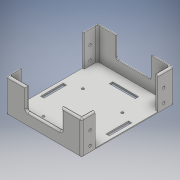
# Autodesk Inventor part: my_body
Saved by Autodesk Inventor 2017.2 (Build 212231000, 231)
## iProperties
Part Number: my_body
Material: Типовые
Document SubType Name: Modeling
Designer: creat
Density: 1 g/cm^3
Appearance: По умолчанию
Author: creat
Autodesk Inventor part; units mm, degrees
ref_plane "YZ Plane" through (0, 0, 0) normal (1, 0, 0) x (0, 1, 0)
ref_plane "XZ Plane" through (0, 0, 0) normal (0, 1, 0) x (-1, 0, 0)
ref_plane "XY Plane" through (0, 0, 0) normal (0, 0, 1) x (1, 0, 0)
sketch "Эскиз1" plane through (0, 0, 0) normal (0, 0, 1) x (1, 0, 0)
  line L0 (0, 12) -> (86, 12)
  line L1 (88, 10) -> (88, -96)
  line L2 (86, -98) -> (0, -98)
  line L3 (-2, -96) -> (-2, 10)
  line L4 (86, -98) -> (86, -96)
  line L5 (86, -96) -> (88, -96)
  arc A0 (-2, -96) -> (0, -98) centre (0, -96) ccw
  arc A1 (0, 12) -> (-2, 10) centre (0, 10) ccw
  arc A2 (88, 10) -> (86, 12) centre (86, 10) ccw
  arc A3 (86, -98) -> (88, -96) centre (86, -96) ccw
  point P0 (0, 0)
  point P1 (88, -98)
  point P2 (88, 12)
  point P3 (-2, -98)
  dimension "d0" = 90
  dimension "d1" = 110
  dimension "d4" = 2
  dimension "d5" = 2
  dimension "d10" = 2
  constraints: 12 end point, 8 point on circle, 8 tangent, 6 point on line, 4 centre point, 3 equal radius, 2 parallel, 1 horizontal, 1 perpendicular
  measures "d0" distance of point (88, -98) point (-2, -98)
  measures "d1" distance of point (88, 12) point (88, -98)
  measures "d4" distance of L4.end L5.end
  measures "d5" distance of L4.start L4.end
  measures "d10" radius of A0
extrude "Выдавливание1" add sketch "Эскиз1" along normal blind 40
sketch "Эскиз2" plane through (0, 0, 40) normal (0, 0, 1) x (1, 0, 0)
  line L0 (2, 9) -> (83.6156, 9)
  line L1 (85.6156, 7) -> (85.6156, -93.4907)
  line L2 (83.6156, -95.4907) -> (2, -95.4907)
  line L3 (0, -93.4907) -> (0, 7)
  arc A0 (83.6156, -95.4907) -> (85.6156, -93.4907) centre (83.6156, -93.4907) ccw
  arc A1 (0, -93.4907) -> (2, -95.4907) centre (2, -93.4907) ccw
  circle A2 centre (23.0817, -76.0567) radius 1.3003
  circle A3 centre (18, -24) radius 1.4794
  circle A4 centre (66.2724, -25.2355) radius 1.3051
  circle A5 centre (50.9777, -76.0071) radius 1.4879
  arc A6 (85.6156, 7) -> (83.6156, 9) centre (83.6156, 7) ccw
  arc A7 (2, 9) -> (0, 7) centre (2, 7) ccw
  point P0 (0, 0)
  point P1 (85.6156, -95.4907)
  point P2 (85.6156, 7.0453)
  point P3 (0, -95.4907)
  point P4 (85.6156, 9)
  point P5 (85.6156, -1.9999)
  dimension "d37" = 2
  constraints: 8 centre point, 8 end point, 8 point on circle, 8 point on line, 7 tangent, 1 equal radius, 1 horizontal, 1 parallel, 1 perpendicular
  measures "d37" radius of A6
extrude "Выдавливание2" cut sketch "Эскиз2" against normal blind 38 contours L0 A6 L1 A0 L2 A1 L3 A7 | A2 | A3 | A4 | A5
sketch "Эскиз3" plane through (88, -96, 0) normal (1, 0, 0) x (0, 0, -1)
  circle A0 centre (-23.5, 8) radius 1.5
  circle A1 centre (-7.5, 8) radius 1.5
  circle A2 centre (-23.5, 96) radius 1.5
  circle A3 centre (-7.5, 96) radius 1.5
  point P0 (0, 96)
  dimension "d15" = 3
  dimension "d16" = 3
  dimension "d17" = 3
  dimension "d18" = 3
  constraints: 4 centre point
  measures "d15" diameter of A0
  measures "d16" diameter of A1
  measures "d17" diameter of A2
  measures "d18" diameter of A3
extrude "Выдавливание3" cut sketch "Эскиз3" against normal blind 98.25
sketch "Эскиз4" plane through (0, -98, 0) normal (0, -1, 0) x (1, 0, 0)
  line L0 (22, 40) -> (64, 40)
  line L1 (64, 40) -> (64, 17)
  line L2 (62, 15) -> (24, 15)
  line L3 (22, 17) -> (22, 40)
  arc A0 (22, 17) -> (24, 15) centre (24, 17) ccw
  arc A1 (62, 15) -> (64, 17) centre (62, 17) ccw
  point P0 (0, 0)
  point P1 (64, 15)
  point P2 (22, 15)
  dimension "d21" = 42
  dimension "d22" = 25
  dimension "d25" = 2
  constraints: 8 end point, 4 point on circle, 4 point on line, 4 tangent, 2 centre point, 2 parallel, 1 equal radius, 1 horizontal, 1 perpendicular
  measures "d21" distance of point (64, 15) point (22, 15)
  measures "d22" distance of L0.end point (64, 15)
  measures "d25" radius of A0
extrude "Выдавливание4" cut sketch "Эскиз4" against normal blind 116.5
fillet "Сопряжение1" radius 2 20 edges at (-1.4142, -97.4142, 40) (-2, -43, 40) (-1.4142, 11.4142, 40) (11, 12, 40) (11, -98, 40) (22.5858, -98, 15.5858) (43, -98, 15) (63.4142, -98, 15.5858) (64, -98, 28.5) (22, -98, 28.5) (87.4142, -97.4142, 40) (88, -43, 40) (87.4142, 11.4142, 40) (75, 12, 40) (75, -98, 40) (63.4142, 12, 15.5858) (64, 12, 28.5) (22.5858, 12, 15.5858) (22, 12, 28.5) (43, 12, 15)
sketch "Эскиз5" plane through (-2, -96, 0) normal (-1, 0, 0) x (0, 0, 1)
  line L0 (9, 91) -> (40, 91)
  line L1 (40, 91) -> (40, 13)
  line L2 (40, 13) -> (9, 13)
  line L3 (7, 15) -> (7, 89)
  arc A0 (9, 91) -> (7, 89) centre (9, 89) ccw
  arc A1 (7, 15) -> (9, 13) centre (9, 15) ccw
  point P0 (0, 96)
  dimension "d27" = 2
  constraints: 8 end point, 4 point on circle, 2 centre point, 2 parallel, 2 tangent, 1 equal radius, 1 horizontal, 1 perpendicular
  measures "d27" radius of A0
extrude "Выдавливание5" [suppressed]
fillet "Сопряжение2" radius 1 8 edges at (-1.4142, 11.4142, 0) (43, 12, 0) (87.4142, 11.4142, 0) (88, -43, 0) (87.4142, -97.4142, 0) (43, -98, 0) (-1.4142, -97.4142, 0) (-2, -43, 0)
fillet "Сопряжение3" [suppressed]
sketch "Эскиз6" plane through (0, 0, 0) normal (0, 0, -1) x (-1, 0, 0)
  line L0 (-2, -34) -> (-6, -34)
  line L1 (-6, -34) -> (-6, -61)
  line L2 (-6, -61) -> (-2, -61)
  line L3 (-2, -61) -> (-2, -34)
  line L4 (-80, -34) -> (-84, -34)
  line L5 (-84, -34) -> (-84, -61)
  line L6 (-84, -61) -> (-80, -61)
  line L7 (-80, -61) -> (-80, -34)
  line L8 (-27, -90) -> (-58, -90)
  line L9 (-58, -90) -> (-58, -94)
  line L10 (-58, -94) -> (-27, -94)
  line L11 (-27, -94) -> (-27, -90)
  line L12 (-30, -3) -> (-61, -3)
  line L13 (-61, -3) -> (-61, -7)
  line L14 (-61, -7) -> (-30, -7)
  line L15 (-30, -7) -> (-30, -3)
  point P0 (0, 0)
  constraints: 32 end point, 8 parallel, 4 horizontal, 4 perpendicular
extrude "Выдавливание6" cut sketch "Эскиз6" against normal blind 2.75
sketch "Эскиз7" plane through (0, 0, 2) normal (0, 0, 1) x (1, 0, 0)
  line L0 (69.5594, -14.0478) -> (69.7922, -14.1325)
  line L1 (70.1519, -14.5133) -> (70.2577, -14.7461)
  line L2 (70.0038, -14.3017) -> (70.1519, -14.5133)
  line L3 (69.7922, -14.1325) -> (70.0038, -14.3017)
  line L4 (70.3, -78.4776) -> (68.7765, -80.001)
  line L5 (69.2844, -14.0055) -> (69.5594, -14.0478)
  line L6 (17.9945, -14.0055) -> (69.2844, -14.0055)
  line L7 (17.7406, -14.0478) -> (17.9945, -14.0055)
  line L8 (17.5078, -14.1325) -> (17.7406, -14.0478)
  line L9 (17.2962, -14.3017) -> (17.5078, -14.1325)
  line L10 (17.127, -14.5133) -> (17.2962, -14.3017)
  line L11 (17.0423, -14.7461) -> (17.127, -14.5133)
  line L12 (17, -15) -> (17.0423, -14.7461)
  line L13 (17, -79.0066) -> (17, -15)
  line L14 (17.0423, -79.2605) -> (17, -79.0066)
  line L15 (17.127, -79.4932) -> (17.0423, -79.2605)
  line L16 (17.2962, -79.7048) -> (17.127, -79.4932)
  line L17 (17.5078, -79.8741) -> (17.2962, -79.7048)
  line L18 (17.7406, -79.9587) -> (17.5078, -79.8741)
  line L19 (17.9945, -80.001) -> (17.7406, -79.9587)
  line L20 (19.5391, -80.001) -> (17.9945, -80.001)
  line L21 (22.0782, -82.5401) -> (19.5391, -80.001)
  line L22 (54.8115, -82.5401) -> (22.0782, -82.5401)
  line L23 (57.3506, -80.001) -> (54.8115, -82.5401)
  line L24 (68.7765, -80.001) -> (57.3506, -80.001)
  line L25 (70.3, -15) -> (70.3, -78.4776)
  line L26 (70.2577, -14.7461) -> (70.3, -15)
  line L27 (66.1538, -29.2963) -> (66.1567, -29.3523)
  line L28 (66.1567, -29.3523) -> (66.1616, -29.4082)
  line L29 (66.1616, -29.4082) -> (66.1684, -29.4639)
  line L30 (66.1684, -29.4639) -> (66.1772, -29.5194)
  line L31 (66.1772, -29.5194) -> (66.1879, -29.5745)
  line L32 (66.1879, -29.5745) -> (66.2006, -29.6292)
  line L33 (66.2006, -29.6292) -> (66.2151, -29.6834)
  line L34 (66.2151, -29.6834) -> (66.2315, -29.7371)
  line L35 (66.2315, -29.7371) -> (66.2498, -29.7901)
  line L36 (66.2498, -29.7901) -> (66.2699, -29.8425)
  line L37 (66.2699, -29.8425) -> (66.2918, -29.8942)
  line L38 (66.2918, -29.8942) -> (66.3155, -29.9451)
  line L39 (66.3155, -29.9451) -> (66.341, -29.9951)
  line L40 (66.341, -29.9951) -> (66.3682, -30.0442)
  line L41 (66.3682, -30.0442) -> (66.3972, -30.0923)
  line L42 (66.3972, -30.0923) -> (66.4277, -30.1394)
  line L43 (66.4277, -30.1394) -> (66.4599, -30.1854)
  line L44 (66.4599, -30.1854) -> (66.4937, -30.2302)
  line L45 (66.4937, -30.2302) -> (66.529, -30.2738)
  line L46 (66.529, -30.2738) -> (66.5658, -30.3162)
  line L47 (66.5658, -30.3162) -> (66.6041, -30.3572)
  line L48 (66.6041, -30.3572) -> (66.6438, -30.3969)
  line L49 (66.6438, -30.3969) -> (66.6849, -30.4352)
  line L50 (66.6849, -30.4352) -> (66.7272, -30.472)
  line L51 (66.7272, -30.472) -> (66.7709, -30.5073)
  line L52 (66.7709, -30.5073) -> (66.8157, -30.5411)
  line L53 (66.8157, -30.5411) -> (66.8617, -30.5733)
  line L54 (66.8617, -30.5733) -> (66.9087, -30.6039)
  line L55 (66.9087, -30.6039) -> (66.9568, -30.6328)
  line L56 (66.9568, -30.6328) -> (67.0059, -30.66)
  line L57 (67.0059, -30.66) -> (67.056, -30.6855)
  line L58 (67.056, -30.6855) -> (67.1068, -30.7092)
  line L59 (67.1068, -30.7092) -> (67.1585, -30.7311)
  line L60 (67.1585, -30.7311) -> (67.2109, -30.7513)
  line L61 (67.2109, -30.7513) -> (67.264, -30.7695)
  line L62 (67.264, -30.7695) -> (67.3176, -30.7859)
  line L63 (67.3176, -30.7859) -> (67.3719, -30.8005)
  line L64 (67.3719, -30.8005) -> (67.4266, -30.8131)
  line L65 (67.4266, -30.8131) -> (67.4817, -30.8238)
  line L66 (67.4817, -30.8238) -> (67.5371, -30.8326)
  line L67 (67.5371, -30.8326) -> (67.5928, -30.8394)
  line L68 (67.5928, -30.8394) -> (67.6487, -30.8443)
  line L69 (67.6487, -30.8443) -> (67.7048, -30.8473)
  line L70 (67.7048, -30.8473) -> (67.7609, -30.8482)
  line L71 (67.7609, -30.8482) -> (67.8166, -30.8473)
  line L72 (67.8166, -30.8473) -> (67.8722, -30.8444)
  line L73 (67.8722, -30.8444) -> (67.9278, -30.8396)
  line L74 (67.9278, -30.8396) -> (67.9831, -30.8328)
  line L75 (67.9831, -30.8328) -> (68.0381, -30.8242)
  line L76 (68.0381, -30.8242) -> (68.0928, -30.8136)
  line L77 (68.0928, -30.8136) -> (68.1471, -30.8012)
  line L78 (68.1471, -30.8012) -> (68.201, -30.7868)
  line L79 (68.201, -30.7868) -> (68.2543, -30.7707)
  line L80 (68.2543, -30.7707) -> (68.307, -30.7527)
  line L81 (68.307, -30.7527) -> (68.3591, -30.7328)
  line L82 (68.3591, -30.7328) -> (68.4104, -30.7112)
  line L83 (68.4104, -30.7112) -> (68.461, -30.6878)
  line L84 (68.461, -30.6878) -> (68.5107, -30.6627)
  line L85 (68.5107, -30.6627) -> (68.5596, -30.6359)
  line L86 (68.5596, -30.6359) -> (68.6075, -30.6074)
  line L87 (68.6075, -30.6074) -> (68.6543, -30.5772)
  line L88 (68.6543, -30.5772) -> (68.7001, -30.5455)
  line L89 (68.7001, -30.5455) -> (68.7448, -30.5121)
  line L90 (68.7448, -30.5121) -> (68.7882, -30.4773)
  line L91 (68.7882, -30.4773) -> (68.8305, -30.441)
  line L92 (68.8305, -30.441) -> (68.8714, -30.4032)
  line L93 (68.8714, -30.4032) -> (68.9111, -30.364)
  line L94 (68.9111, -30.364) -> (68.9493, -30.3235)
  line L95 (68.9493, -30.3235) -> (68.9861, -30.2817)
  line L96 (68.9861, -30.2817) -> (69.0215, -30.2386)
  line L97 (69.0215, -30.2386) -> (69.0553, -30.1943)
  line L98 (69.0553, -30.1943) -> (69.0876, -30.1489)
  line L99 (69.0876, -30.1489) -> (69.1183, -30.1024)
  line L100 (69.1183, -30.1024) -> (69.1473, -30.0549)
  line L101 (69.1473, -30.0549) -> (69.1747, -30.0064)
  line L102 (69.1747, -30.0064) -> (69.2004, -29.9569)
  line L103 (69.2004, -29.9569) -> (69.2244, -29.9066)
  line L104 (69.2244, -29.9066) -> (69.2466, -29.8555)
  line L105 (69.2466, -29.8555) -> (69.267, -29.8037)
  line L106 (69.267, -29.8037) -> (69.2856, -29.7512)
  line L107 (69.2856, -29.7512) -> (69.3024, -29.698)
  line L108 (69.3024, -29.698) -> (69.3174, -29.6444)
  line L109 (69.3174, -29.6444) -> (69.3304, -29.5902)
  line L110 (69.3304, -29.5902) -> (69.3416, -29.5356)
  line L111 (69.3416, -29.5356) -> (69.3509, -29.4807)
  line L112 (69.3509, -29.4807) -> (69.3583, -29.4255)
  line L113 (69.3583, -29.4255) -> (69.3637, -29.37)
  line L114 (69.3637, -29.37) -> (69.3673, -29.3144)
  line L115 (69.3673, -29.3144) -> (69.3689, -29.2587)
  line L116 (69.3689, -29.2587) -> (69.3686, -29.203)
  line L117 (69.3686, -29.203) -> (69.3663, -29.1473)
  line L118 (69.3663, -29.1473) -> (69.3621, -29.0918)
  line L119 (66.1528, -29.2401) -> (66.1538, -29.2963)
  line L120 (69.356, -29.0364) -> (69.348, -28.9812)
  line L121 (69.348, -28.9812) -> (69.3381, -28.9264)
  line L122 (69.3381, -28.9264) -> (69.3263, -28.872)
  line L123 (69.3263, -28.872) -> (69.3126, -28.818)
  line L124 (69.3126, -28.818) -> (69.297, -28.7644)
  line L125 (69.297, -28.7644) -> (69.2796, -28.7115)
  line L126 (69.2796, -28.7115) -> (69.2604, -28.6592)
  line L127 (69.2604, -28.6592) -> (69.2394, -28.6076)
  line L128 (69.2394, -28.6076) -> (69.2166, -28.5568)
  line L129 (69.2166, -28.5568) -> (69.192, -28.5068)
  line L130 (69.192, -28.5068) -> (69.1658, -28.4576)
  line L131 (69.1658, -28.4576) -> (69.1378, -28.4094)
  line L132 (69.1378, -28.4094) -> (69.1082, -28.3622)
  line L133 (69.1082, -28.3622) -> (69.077, -28.3161)
  line L134 (69.077, -28.3161) -> (69.0442, -28.271)
  line L135 (69.0442, -28.271) -> (69.0098, -28.2272)
  line L136 (69.0098, -28.2272) -> (68.974, -28.1845)
  line L137 (68.974, -28.1845) -> (68.9367, -28.1431)
  line L138 (68.9367, -28.1431) -> (68.898, -28.103)
  line L139 (68.898, -28.103) -> (68.8579, -28.0643)
  line L140 (68.8579, -28.0643) -> (68.8165, -28.027)
  line L141 (68.8165, -28.027) -> (68.7739, -27.9912)
  line L142 (68.7739, -27.9912) -> (68.73, -27.9568)
  line L143 (68.73, -27.9568) -> (68.685, -27.924)
  line L144 (68.685, -27.924) -> (68.6388, -27.8928)
  line L145 (68.6388, -27.8928) -> (68.5916, -27.8632)
  line L146 (68.5916, -27.8632) -> (68.5434, -27.8353)
  line L147 (68.5434, -27.8353) -> (68.4943, -27.809)
  line L148 (68.4943, -27.809) -> (68.4442, -27.7845)
  line L149 (68.4442, -27.7845) -> (68.3934, -27.7617)
  line L150 (68.3934, -27.7617) -> (68.3418, -27.7406)
  line L151 (68.3418, -27.7406) -> (68.2895, -27.7214)
  line L152 (68.2895, -27.7214) -> (68.2366, -27.704)
  line L153 (68.2366, -27.704) -> (68.1831, -27.6884)
  line L154 (68.1831, -27.6884) -> (68.1291, -27.6748)
  line L155 (68.1291, -27.6748) -> (68.0746, -27.6629)
  line L156 (68.0746, -27.6629) -> (68.0198, -27.653)
  line L157 (68.0198, -27.653) -> (67.9647, -27.645)
  line L158 (67.9647, -27.645) -> (67.9093, -27.6389)
  line L159 (67.9093, -27.6389) -> (67.8537, -27.6347)
  line L160 (67.8537, -27.6347) -> (67.798, -27.6325)
  line L161 (67.798, -27.6325) -> (67.7423, -27.6321)
  line L162 (67.7423, -27.6321) -> (67.6866, -27.6338)
  line L163 (67.6866, -27.6338) -> (67.631, -27.6373)
  line L164 (67.631, -27.6373) -> (67.5756, -27.6428)
  line L165 (67.5756, -27.6428) -> (67.5203, -27.6501)
  line L166 (67.5203, -27.6501) -> (67.4654, -27.6594)
  line L167 (67.4654, -27.6594) -> (67.4108, -27.6706)
  line L168 (67.4108, -27.6706) -> (67.3567, -27.6837)
  line L169 (67.3567, -27.6837) -> (67.303, -27.6986)
  line L170 (67.303, -27.6986) -> (67.2499, -27.7154)
  line L171 (67.2499, -27.7154) -> (67.1973, -27.734)
  line L172 (67.1973, -27.734) -> (67.1455, -27.7544)
  line L173 (67.1455, -27.7544) -> (67.0944, -27.7767)
  line L174 (67.0944, -27.7767) -> (67.0441, -27.8006)
  line L175 (67.0441, -27.8006) -> (66.9947, -27.8263)
  line L176 (66.9947, -27.8263) -> (66.9461, -27.8537)
  line L177 (66.9461, -27.8537) -> (66.8986, -27.8828)
  line L178 (66.8986, -27.8828) -> (66.8521, -27.9135)
  line L179 (66.8521, -27.9135) -> (66.8067, -27.9457)
  line L180 (66.8067, -27.9457) -> (66.7624, -27.9796)
  line L181 (66.7624, -27.9796) -> (66.7193, -28.0149)
  line L182 (66.7193, -28.0149) -> (66.6775, -28.0517)
  line L183 (66.6775, -28.0517) -> (66.637, -28.09)
  line L184 (66.637, -28.09) -> (66.5978, -28.1296)
  line L185 (66.5978, -28.1296) -> (66.5601, -28.1706)
  line L186 (66.5601, -28.1706) -> (66.5237, -28.2128)
  line L187 (66.5237, -28.2128) -> (66.4889, -28.2563)
  line L188 (66.4889, -28.2563) -> (66.4556, -28.3009)
  line L189 (66.4556, -28.3009) -> (66.4238, -28.3467)
  line L190 (66.4238, -28.3467) -> (66.3937, -28.3936)
  line L191 (66.3937, -28.3936) -> (66.3652, -28.4415)
  line L192 (66.3652, -28.4415) -> (66.3383, -28.4903)
  line L193 (66.3383, -28.4903) -> (66.3132, -28.54)
  line L194 (66.3132, -28.54) -> (66.2898, -28.5906)
  line L195 (66.2898, -28.5906) -> (66.2682, -28.6419)
  line L196 (66.2682, -28.6419) -> (66.2484, -28.694)
  line L197 (66.2484, -28.694) -> (66.2304, -28.7467)
  line L198 (66.2304, -28.7467) -> (66.2142, -28.8001)
  line L199 (66.2142, -28.8001) -> (66.1999, -28.8539)
  line L200 (66.1999, -28.8539) -> (66.1874, -28.9082)
  line L201 (66.1874, -28.9082) -> (66.1769, -28.9629)
  line L202 (66.1769, -28.9629) -> (66.1682, -29.018)
  line L203 (66.1682, -29.018) -> (66.1615, -29.0733)
  line L204 (66.1615, -29.0733) -> (66.1567, -29.1288)
  line L205 (66.1567, -29.1288) -> (66.1538, -29.1844)
  line L206 (66.1538, -29.1844) -> (66.1528, -29.2401)
  line L207 (69.3621, -29.0918) -> (69.356, -29.0364)
  line L208 (50.9182, -80.001) -> (50.9192, -80.0572)
  line L209 (50.9192, -80.0572) -> (50.9221, -80.1132)
  line L210 (50.9221, -80.1132) -> (50.927, -80.1691)
  line L211 (50.927, -80.1691) -> (50.9338, -80.2248)
  line L212 (50.9338, -80.2248) -> (50.9426, -80.2803)
  line L213 (50.9426, -80.2803) -> (50.9533, -80.3354)
  line L214 (50.9533, -80.3354) -> (50.9659, -80.3901)
  line L215 (50.9659, -80.3901) -> (50.9805, -80.4443)
  line L216 (50.9805, -80.4443) -> (50.9969, -80.498)
  line L217 (50.9969, -80.498) -> (51.0152, -80.551)
  line L218 (51.0152, -80.551) -> (51.0353, -80.6034)
  line L219 (51.0353, -80.6034) -> (51.0572, -80.6551)
  line L220 (51.0572, -80.6551) -> (51.0809, -80.706)
  line L221 (51.0809, -80.706) -> (51.1064, -80.756)
  line L222 (51.1064, -80.756) -> (51.1336, -80.8051)
  line L223 (51.1336, -80.8051) -> (51.1625, -80.8532)
  line L224 (51.1625, -80.8532) -> (51.1931, -80.9003)
  line L225 (51.1931, -80.9003) -> (51.2253, -80.9462)
  line L226 (51.2253, -80.9462) -> (51.2591, -80.9911)
  line L227 (51.2591, -80.9911) -> (51.2944, -81.0347)
  line L228 (51.2944, -81.0347) -> (51.3312, -81.0771)
  line L229 (51.3312, -81.0771) -> (51.3695, -81.1181)
  line L230 (51.3695, -81.1181) -> (51.4092, -81.1578)
  line L231 (51.4092, -81.1578) -> (51.4503, -81.1961)
  line L232 (51.4503, -81.1961) -> (51.4926, -81.2329)
  line L233 (51.4926, -81.2329) -> (51.5362, -81.2682)
  line L234 (51.5362, -81.2682) -> (51.5811, -81.302)
  line L235 (51.5811, -81.302) -> (51.627, -81.3342)
  line L236 (51.627, -81.3342) -> (51.6741, -81.3648)
  line L237 (51.6741, -81.3648) -> (51.7222, -81.3937)
  line L238 (51.7222, -81.3937) -> (51.7713, -81.4209)
  line L239 (51.7713, -81.4209) -> (51.8213, -81.4464)
  line L240 (51.8213, -81.4464) -> (51.8722, -81.4701)
  line L241 (51.8722, -81.4701) -> (51.9239, -81.492)
  line L242 (51.9239, -81.492) -> (51.9763, -81.5122)
  line L243 (51.9763, -81.5122) -> (52.0294, -81.5304)
  line L244 (52.0294, -81.5304) -> (52.083, -81.5468)
  line L245 (52.083, -81.5468) -> (52.1372, -81.5614)
  line L246 (52.1372, -81.5614) -> (52.1919, -81.574)
  line L247 (52.1919, -81.574) -> (52.247, -81.5847)
  line L248 (52.247, -81.5847) -> (52.3025, -81.5935)
  line L249 (52.3025, -81.5935) -> (52.3582, -81.6003)
  line L250 (52.3582, -81.6003) -> (52.4141, -81.6052)
  line L251 (52.4141, -81.6052) -> (52.4702, -81.6082)
  line L252 (52.4702, -81.6082) -> (52.5263, -81.6091)
  line L253 (52.5263, -81.6091) -> (52.582, -81.6082)
  line L254 (52.582, -81.6082) -> (52.6376, -81.6053)
  line L255 (52.6376, -81.6053) -> (52.6931, -81.6005)
  line L256 (52.6931, -81.6005) -> (52.7484, -81.5937)
  line L257 (52.7484, -81.5937) -> (52.8035, -81.5851)
  line L258 (52.8035, -81.5851) -> (52.8582, -81.5745)
  line L259 (52.8582, -81.5745) -> (52.9125, -81.5621)
  line L260 (52.9125, -81.5621) -> (52.9664, -81.5477)
  line L261 (52.9664, -81.5477) -> (53.0197, -81.5316)
  line L262 (53.0197, -81.5316) -> (53.0724, -81.5136)
  line L263 (53.0724, -81.5136) -> (53.1245, -81.4937)
  line L264 (53.1245, -81.4937) -> (53.1758, -81.4721)
  line L265 (53.1758, -81.4721) -> (53.2264, -81.4487)
  line L266 (53.2264, -81.4487) -> (53.2761, -81.4236)
  line L267 (53.2761, -81.4236) -> (53.325, -81.3968)
  line L268 (53.325, -81.3968) -> (53.3728, -81.3683)
  line L269 (53.3728, -81.3683) -> (53.4197, -81.3381)
  line L270 (53.4197, -81.3381) -> (53.4655, -81.3064)
  line L271 (53.4655, -81.3064) -> (53.5101, -81.273)
  line L272 (53.5101, -81.273) -> (53.5536, -81.2382)
  line L273 (53.5536, -81.2382) -> (53.5959, -81.2019)
  line L274 (53.5959, -81.2019) -> (53.6368, -81.1641)
  line L275 (53.6368, -81.1641) -> (53.6764, -81.1249)
  line L276 (53.6764, -81.1249) -> (53.7147, -81.0844)
  line L277 (53.7147, -81.0844) -> (53.7515, -81.0426)
  line L278 (53.7515, -81.0426) -> (53.7868, -80.9995)
  line L279 (53.7868, -80.9995) -> (53.8207, -80.9552)
  line L280 (53.8207, -80.9552) -> (53.853, -80.9098)
  line L281 (53.853, -80.9098) -> (53.8836, -80.8633)
  line L282 (53.8836, -80.8633) -> (53.9127, -80.8158)
  line L283 (53.9127, -80.8158) -> (53.9401, -80.7673)
  line L284 (53.9401, -80.7673) -> (53.9658, -80.7178)
  line L285 (53.9658, -80.7178) -> (53.9898, -80.6675)
  line L286 (53.9898, -80.6675) -> (54.012, -80.6164)
  line L287 (54.012, -80.6164) -> (54.0324, -80.5646)
  line L288 (54.0324, -80.5646) -> (54.051, -80.5121)
  line L289 (54.051, -80.5121) -> (54.0678, -80.4589)
  line L290 (54.0678, -80.4589) -> (54.0827, -80.4053)
  line L291 (54.0827, -80.4053) -> (54.0958, -80.3511)
  line L292 (54.0958, -80.3511) -> (54.107, -80.2965)
  line L293 (54.107, -80.2965) -> (54.1163, -80.2416)
  line L294 (54.1163, -80.2416) -> (54.1237, -80.1864)
  line L295 (54.1237, -80.1864) -> (54.1291, -80.1309)
  line L296 (54.1291, -80.1309) -> (54.1327, -80.0753)
  line L297 (54.1327, -80.0753) -> (54.1343, -80.0196)
  line L298 (54.1343, -80.0196) -> (54.1339, -79.9639)
  line L299 (54.1339, -79.9639) -> (54.1317, -79.9082)
  line L300 (54.1317, -79.9082) -> (54.1275, -79.8527)
  line L301 (54.1275, -79.8527) -> (54.1214, -79.7973)
  line L302 (54.1214, -79.7973) -> (54.1134, -79.7421)
  line L303 (54.1134, -79.7421) -> (54.1035, -79.6873)
  line L304 (54.1035, -79.6873) -> (54.0917, -79.6329)
  line L305 (54.0917, -79.6329) -> (54.078, -79.5788)
  line L306 (54.078, -79.5788) -> (54.0624, -79.5253)
  line L307 (54.0624, -79.5253) -> (54.045, -79.4724)
  line L308 (54.045, -79.4724) -> (54.0258, -79.4201)
  line L309 (54.0258, -79.4201) -> (54.0048, -79.3685)
  line L310 (54.0048, -79.3685) -> (53.982, -79.3177)
  line L311 (53.982, -79.3177) -> (53.9574, -79.2677)
  line L312 (53.9574, -79.2677) -> (53.9312, -79.2185)
  line L313 (53.9312, -79.2185) -> (53.9032, -79.1703)
  line L314 (53.9032, -79.1703) -> (53.8736, -79.1231)
  line L315 (53.8736, -79.1231) -> (53.8424, -79.077)
  line L316 (53.8424, -79.077) -> (53.8096, -79.0319)
  line L317 (53.8096, -79.0319) -> (53.7752, -78.9881)
  line L318 (53.7752, -78.9881) -> (53.7394, -78.9454)
  line L319 (53.7394, -78.9454) -> (53.7021, -78.904)
  line L320 (53.7021, -78.904) -> (53.6634, -78.8639)
  line L321 (53.6634, -78.8639) -> (53.6233, -78.8252)
  line L322 (53.6233, -78.8252) -> (53.5819, -78.7879)
  line L323 (53.5819, -78.7879) -> (53.5393, -78.7521)
  line L324 (53.5393, -78.7521) -> (53.4954, -78.7177)
  line L325 (53.4954, -78.7177) -> (53.4503, -78.6849)
  line L326 (53.4503, -78.6849) -> (53.4042, -78.6537)
  line L327 (53.4042, -78.6537) -> (53.357, -78.6241)
  line L328 (53.357, -78.6241) -> (53.3088, -78.5962)
  line L329 (53.3088, -78.5962) -> (53.2596, -78.5699)
  line L330 (53.2596, -78.5699) -> (53.2096, -78.5453)
  line L331 (53.2096, -78.5453) -> (53.1588, -78.5225)
  line L332 (53.1588, -78.5225) -> (53.1072, -78.5015)
  line L333 (53.1072, -78.5015) -> (53.0549, -78.4823)
  line L334 (53.0549, -78.4823) -> (53.002, -78.4649)
  line L335 (53.002, -78.4649) -> (52.9485, -78.4493)
  line L336 (52.9485, -78.4493) -> (52.8945, -78.4356)
  line L337 (52.8945, -78.4356) -> (52.84, -78.4238)
  line L338 (52.84, -78.4238) -> (52.7852, -78.4139)
  line L339 (52.7852, -78.4139) -> (52.73, -78.4059)
  line L340 (52.73, -78.4059) -> (52.6747, -78.3998)
  line L341 (52.6747, -78.3998) -> (52.6191, -78.3956)
  line L342 (52.6191, -78.3956) -> (52.5634, -78.3934)
  line L343 (52.5634, -78.3934) -> (52.5077, -78.393)
  line L344 (52.5077, -78.393) -> (52.452, -78.3946)
  line L345 (52.452, -78.3946) -> (52.3964, -78.3982)
  line L346 (52.3964, -78.3982) -> (52.341, -78.4036)
  line L347 (52.341, -78.4036) -> (52.2857, -78.411)
  line L348 (52.2857, -78.411) -> (52.2308, -78.4203)
  line L349 (52.2308, -78.4203) -> (52.1762, -78.4315)
  line L350 (52.1762, -78.4315) -> (52.122, -78.4446)
  line L351 (52.122, -78.4446) -> (52.0684, -78.4595)
  line L352 (52.0684, -78.4595) -> (52.0152, -78.4763)
  line L353 (52.0152, -78.4763) -> (51.9627, -78.4949)
  line L354 (51.9627, -78.4949) -> (51.9109, -78.5153)
  line L355 (51.9109, -78.5153) -> (51.8598, -78.5376)
  line L356 (51.8598, -78.5376) -> (51.8095, -78.5615)
  line L357 (51.8095, -78.5615) -> (51.7601, -78.5872)
  line L358 (51.7601, -78.5872) -> (51.7115, -78.6146)
  line L359 (51.7115, -78.6146) -> (51.664, -78.6437)
  line L360 (51.664, -78.6437) -> (51.6175, -78.6744)
  line L361 (51.6175, -78.6744) -> (51.5721, -78.7066)
  line L362 (51.5721, -78.7066) -> (51.5278, -78.7405)
  line L363 (51.5278, -78.7405) -> (51.4847, -78.7758)
  line L364 (51.4847, -78.7758) -> (51.4429, -78.8126)
  line L365 (51.4429, -78.8126) -> (51.4024, -78.8509)
  line L366 (51.4024, -78.8509) -> (51.3632, -78.8905)
  line L367 (51.3632, -78.8905) -> (51.3254, -78.9315)
  line L368 (51.3254, -78.9315) -> (51.2891, -78.9737)
  line L369 (51.2891, -78.9737) -> (51.2543, -79.0172)
  line L370 (51.2543, -79.0172) -> (51.2209, -79.0618)
  line L371 (51.2209, -79.0618) -> (51.1892, -79.1076)
  line L372 (51.1892, -79.1076) -> (51.159, -79.1545)
  line L373 (51.159, -79.1545) -> (51.1305, -79.2024)
  line L374 (51.1305, -79.2024) -> (51.1037, -79.2512)
  line L375 (51.1037, -79.2512) -> (51.0786, -79.3009)
  line L376 (51.0786, -79.3009) -> (51.0552, -79.3515)
  line L377 (51.0552, -79.3515) -> (51.0336, -79.4028)
  line L378 (51.0336, -79.4028) -> (51.0138, -79.4549)
  line L379 (51.0138, -79.4549) -> (50.9957, -79.5076)
  line L380 (50.9957, -79.5076) -> (50.9796, -79.561)
  line L381 (50.9796, -79.561) -> (50.9653, -79.6148)
  line L382 (50.9653, -79.6148) -> (50.9528, -79.6691)
  line L383 (50.9528, -79.6691) -> (50.9423, -79.7238)
  line L384 (50.9423, -79.7238) -> (50.9336, -79.7789)
  line L385 (50.9336, -79.7789) -> (50.9269, -79.8342)
  line L386 (50.9269, -79.8342) -> (50.922, -79.8897)
  line L387 (50.922, -79.8897) -> (50.9191, -79.9453)
  line L388 (50.9191, -79.9453) -> (50.9182, -80.001)
  line L389 (17.931, -27.9706) -> (17.932, -28.0267)
  line L390 (17.932, -28.0267) -> (17.9349, -28.0828)
  line L391 (17.9349, -28.0828) -> (17.9398, -28.1387)
  line L392 (17.9398, -28.1387) -> (17.9467, -28.1944)
  line L393 (17.9467, -28.1944) -> (17.9554, -28.2498)
  line L394 (17.9554, -28.2498) -> (17.9661, -28.3049)
  line L395 (17.9661, -28.3049) -> (17.9788, -28.3596)
  line L396 (17.9788, -28.3596) -> (17.9933, -28.4138)
  line L397 (17.9933, -28.4138) -> (18.0097, -28.4675)
  line L398 (18.0097, -28.4675) -> (18.028, -28.5206)
  line L399 (18.028, -28.5206) -> (18.0481, -28.573)
  line L400 (18.0481, -28.573) -> (18.07, -28.6247)
  line L401 (18.07, -28.6247) -> (18.0938, -28.6755)
  line L402 (18.0938, -28.6755) -> (18.1192, -28.7255)
  line L403 (18.1192, -28.7255) -> (18.1464, -28.7746)
  line L404 (18.1464, -28.7746) -> (18.1754, -28.8227)
  line L405 (18.1754, -28.8227) -> (18.2059, -28.8698)
  line L406 (18.2059, -28.8698) -> (18.2381, -28.9158)
  line L407 (18.2381, -28.9158) -> (18.2719, -28.9606)
  line L408 (18.2719, -28.9606) -> (18.3072, -29.0042)
  line L409 (18.3072, -29.0042) -> (18.3441, -29.0466)
  line L410 (18.3441, -29.0466) -> (18.3823, -29.0877)
  line L411 (18.3823, -29.0877) -> (18.422, -29.1274)
  line L412 (18.422, -29.1274) -> (18.4631, -29.1656)
  line L413 (18.4631, -29.1656) -> (18.5054, -29.2025)
  line L414 (18.5054, -29.2025) -> (18.5491, -29.2378)
  line L415 (18.5491, -29.2378) -> (18.5939, -29.2716)
  line L416 (18.5939, -29.2716) -> (18.6399, -29.3038)
  line L417 (18.6399, -29.3038) -> (18.6869, -29.3343)
  line L418 (18.6869, -29.3343) -> (18.7351, -29.3632)
  line L419 (18.7351, -29.3632) -> (18.7841, -29.3905)
  line L420 (18.7841, -29.3905) -> (18.8342, -29.4159)
  line L421 (18.8342, -29.4159) -> (18.885, -29.4397)
  line L422 (18.885, -29.4397) -> (18.9367, -29.4616)
  line L423 (18.9367, -29.4616) -> (18.9891, -29.4817)
  line L424 (18.9891, -29.4817) -> (19.0422, -29.5)
  line L425 (19.0422, -29.5) -> (19.0959, -29.5164)
  line L426 (19.0959, -29.5164) -> (19.1501, -29.5309)
  line L427 (19.1501, -29.5309) -> (19.2048, -29.5435)
  line L428 (19.2048, -29.5435) -> (19.2599, -29.5543)
  line L429 (19.2599, -29.5543) -> (19.3153, -29.563)
  line L430 (19.3153, -29.563) -> (19.371, -29.5699)
  line L431 (19.371, -29.5699) -> (19.4269, -29.5748)
  line L432 (19.4269, -29.5748) -> (19.483, -29.5777)
  line L433 (19.483, -29.5777) -> (19.5391, -29.5787)
  line L434 (19.5391, -29.5787) -> (19.5948, -29.5777)
  line L435 (19.5948, -29.5777) -> (19.6505, -29.5748)
  line L436 (19.6505, -29.5748) -> (19.706, -29.57)
  line L437 (19.706, -29.57) -> (19.7613, -29.5633)
  line L438 (19.7613, -29.5633) -> (19.8163, -29.5546)
  line L439 (19.8163, -29.5546) -> (19.871, -29.5441)
  line L440 (19.871, -29.5441) -> (19.9253, -29.5316)
  line L441 (19.9253, -29.5316) -> (19.9792, -29.5173)
  line L442 (19.9792, -29.5173) -> (20.0325, -29.5011)
  line L443 (20.0325, -29.5011) -> (20.0852, -29.4831)
  line L444 (20.0852, -29.4831) -> (20.1373, -29.4633)
  line L445 (20.1373, -29.4633) -> (20.1886, -29.4417)
  line L446 (20.1886, -29.4417) -> (20.2392, -29.4183)
  line L447 (20.2392, -29.4183) -> (20.289, -29.3932)
  line L448 (20.289, -29.3932) -> (20.3378, -29.3663)
  line L449 (20.3378, -29.3663) -> (20.3857, -29.3378)
  line L450 (20.3857, -29.3378) -> (20.4325, -29.3077)
  line L451 (20.4325, -29.3077) -> (20.4783, -29.2759)
  line L452 (20.4783, -29.2759) -> (20.523, -29.2426)
  line L453 (20.523, -29.2426) -> (20.5664, -29.2077)
  line L454 (20.5664, -29.2077) -> (20.6087, -29.1714)
  line L455 (20.6087, -29.1714) -> (20.6496, -29.1336)
  line L456 (20.6496, -29.1336) -> (20.6893, -29.0945)
  line L457 (20.6893, -29.0945) -> (20.7275, -29.054)
  line L458 (20.7275, -29.054) -> (20.7643, -29.0121)
  line L459 (20.7643, -29.0121) -> (20.7997, -28.9691)
  line L460 (20.7997, -28.9691) -> (20.8335, -28.9248)
  line L461 (20.8335, -28.9248) -> (20.8658, -28.8794)
  line L462 (20.8658, -28.8794) -> (20.8965, -28.8329)
  line L463 (20.8965, -28.8329) -> (20.9255, -28.7853)
  line L464 (20.9255, -28.7853) -> (20.9529, -28.7368)
  line L465 (20.9529, -28.7368) -> (20.9786, -28.6874)
  line L466 (20.9786, -28.6874) -> (21.0026, -28.6371)
  line L467 (21.0026, -28.6371) -> (21.0248, -28.586)
  line L468 (21.0248, -28.586) -> (21.0452, -28.5341)
  line L469 (21.0452, -28.5341) -> (21.0638, -28.4816)
  line L470 (21.0638, -28.4816) -> (21.0806, -28.4285)
  line L471 (21.0806, -28.4285) -> (21.0956, -28.3748)
  line L472 (21.0956, -28.3748) -> (21.1086, -28.3207)
  line L473 (21.1086, -28.3207) -> (21.1198, -28.2661)
  line L474 (21.1198, -28.2661) -> (21.1291, -28.2111)
  line L475 (21.1291, -28.2111) -> (21.1365, -28.1559)
  line L476 (21.1365, -28.1559) -> (21.1419, -28.1005)
  line L477 (21.1419, -28.1005) -> (21.1455, -28.0449)
  line L478 (21.1455, -28.0449) -> (21.1471, -27.9892)
  line L479 (21.1471, -27.9892) -> (21.1468, -27.9334)
  line L480 (21.1468, -27.9334) -> (21.1445, -27.8778)
  line L481 (21.1445, -27.8778) -> (21.1403, -27.8222)
  line L482 (21.1403, -27.8222) -> (21.1342, -27.7668)
  line L483 (21.1342, -27.7668) -> (21.1262, -27.7117)
  line L484 (21.1262, -27.7117) -> (21.1163, -27.6569)
  line L485 (21.1163, -27.6569) -> (21.1045, -27.6024)
  line L486 (21.1045, -27.6024) -> (21.0908, -27.5484)
  line L487 (21.0908, -27.5484) -> (21.0752, -27.4949)
  line L488 (21.0752, -27.4949) -> (21.0578, -27.442)
  line L489 (21.0578, -27.442) -> (21.0386, -27.3897)
  line L490 (21.0386, -27.3897) -> (21.0176, -27.3381)
  line L491 (21.0176, -27.3381) -> (20.9948, -27.2872)
  line L492 (20.9948, -27.2872) -> (20.9702, -27.2372)
  line L493 (20.9702, -27.2372) -> (20.944, -27.1881)
  line L494 (20.944, -27.1881) -> (20.916, -27.1399)
  line L495 (20.916, -27.1399) -> (20.8864, -27.0927)
  line L496 (20.8864, -27.0927) -> (20.8552, -27.0465)
  line L497 (20.8552, -27.0465) -> (20.8224, -27.0015)
  line L498 (20.8224, -27.0015) -> (20.7881, -26.9576)
  line L499 (20.7881, -26.9576) -> (20.7522, -26.915)
  line L500 (20.7522, -26.915) -> (20.7149, -26.8736)
  line L501 (20.7149, -26.8736) -> (20.6762, -26.8335)
  line L502 (20.6762, -26.8335) -> (20.6361, -26.7948)
  line L503 (20.6361, -26.7948) -> (20.5947, -26.7575)
  line L504 (20.5947, -26.7575) -> (20.5521, -26.7216)
  line L505 (20.5521, -26.7216) -> (20.5082, -26.6873)
  line L506 (20.5082, -26.6873) -> (20.4632, -26.6545)
  line L507 (20.4632, -26.6545) -> (20.417, -26.6233)
  line L508 (20.417, -26.6233) -> (20.3698, -26.5937)
  line L509 (20.3698, -26.5937) -> (20.3216, -26.5657)
  line L510 (20.3216, -26.5657) -> (20.2725, -26.5394)
  line L511 (20.2725, -26.5394) -> (20.2225, -26.5149)
  line L512 (20.2225, -26.5149) -> (20.1716, -26.4921)
  line L513 (20.1716, -26.4921) -> (20.12, -26.4711)
  line L514 (20.12, -26.4711) -> (20.0677, -26.4519)
  line L515 (20.0677, -26.4519) -> (20.0148, -26.4345)
  line L516 (20.0148, -26.4345) -> (19.9613, -26.4189)
  line L517 (19.9613, -26.4189) -> (19.9073, -26.4052)
  line L518 (19.9073, -26.4052) -> (19.8528, -26.3934)
  line L519 (19.8528, -26.3934) -> (19.798, -26.3835)
  line L520 (19.798, -26.3835) -> (19.7429, -26.3754)
  line L521 (19.7429, -26.3754) -> (19.6875, -26.3693)
  line L522 (19.6875, -26.3693) -> (19.6319, -26.3652)
  line L523 (19.6319, -26.3652) -> (19.5762, -26.3629)
  line L524 (19.5762, -26.3629) -> (19.5205, -26.3626)
  line L525 (19.5205, -26.3626) -> (19.4648, -26.3642)
  line L526 (19.4648, -26.3642) -> (19.4092, -26.3677)
  line L527 (19.4092, -26.3677) -> (19.3538, -26.3732)
  line L528 (19.3538, -26.3732) -> (19.2986, -26.3806)
  line L529 (19.2986, -26.3806) -> (19.2436, -26.3899)
  line L530 (19.2436, -26.3899) -> (19.189, -26.4011)
  line L531 (19.189, -26.4011) -> (19.1349, -26.4141)
  line L532 (19.1349, -26.4141) -> (19.0812, -26.4291)
  line L533 (19.0812, -26.4291) -> (19.0281, -26.4458)
  line L534 (19.0281, -26.4458) -> (18.9755, -26.4645)
  line L535 (18.9755, -26.4645) -> (18.9237, -26.4849)
  line L536 (18.9237, -26.4849) -> (18.8726, -26.5071)
  line L537 (18.8726, -26.5071) -> (18.8223, -26.5311)
  line L538 (18.8223, -26.5311) -> (18.7729, -26.5568)
  line L539 (18.7729, -26.5568) -> (18.7244, -26.5842)
  line L540 (18.7244, -26.5842) -> (18.6768, -26.6132)
  line L541 (18.6768, -26.6132) -> (18.6303, -26.6439)
  line L542 (18.6303, -26.6439) -> (18.5849, -26.6762)
  line L543 (18.5849, -26.6762) -> (18.5406, -26.71)
  line L544 (18.5406, -26.71) -> (18.4976, -26.7454)
  line L545 (18.4976, -26.7454) -> (18.4557, -26.7822)
  line L546 (18.4557, -26.7822) -> (18.4152, -26.8204)
  line L547 (18.4152, -26.8204) -> (18.376, -26.8601)
  line L548 (18.376, -26.8601) -> (18.3383, -26.901)
  line L549 (18.3383, -26.901) -> (18.3019, -26.9433)
  line L550 (18.3019, -26.9433) -> (18.2671, -26.9867)
  line L551 (18.2671, -26.9867) -> (18.2338, -27.0314)
  line L552 (18.2338, -27.0314) -> (18.202, -27.0772)
  line L553 (18.202, -27.0772) -> (18.1719, -27.124)
  line L554 (18.1719, -27.124) -> (18.1434, -27.1719)
  line L555 (18.1434, -27.1719) -> (18.1165, -27.2207)
  line L556 (18.1165, -27.2207) -> (18.0914, -27.2705)
  line L557 (18.0914, -27.2705) -> (18.068, -27.321)
  line L558 (18.068, -27.321) -> (18.0464, -27.3724)
  line L559 (18.0464, -27.3724) -> (18.0266, -27.4245)
  line L560 (18.0266, -27.4245) -> (18.0086, -27.4772)
  line L561 (18.0086, -27.4772) -> (17.9924, -27.5305)
  line L562 (17.9924, -27.5305) -> (17.9781, -27.5844)
  line L563 (17.9781, -27.5844) -> (17.9656, -27.6387)
  line L564 (17.9656, -27.6387) -> (17.9551, -27.6934)
  line L565 (17.9551, -27.6934) -> (17.9464, -27.7484)
  line L566 (17.9464, -27.7484) -> (17.9397, -27.8037)
  line L567 (17.9397, -27.8037) -> (17.9349, -27.8592)
  line L568 (17.9349, -27.8592) -> (17.932, -27.9149)
  line L569 (17.932, -27.9149) -> (17.931, -27.9706)
  line L570 (23.0092, -80.001) -> (23.0102, -80.0572)
  line L571 (23.0102, -80.0572) -> (23.0131, -80.1132)
  line L572 (23.0131, -80.1132) -> (23.018, -80.1691)
  line L573 (23.018, -80.1691) -> (23.0249, -80.2248)
  line L574 (23.0249, -80.2248) -> (23.0336, -80.2803)
  line L575 (23.0336, -80.2803) -> (23.0444, -80.3354)
  line L576 (23.0444, -80.3354) -> (23.057, -80.3901)
  line L577 (23.057, -80.3901) -> (23.0715, -80.4443)
  line L578 (23.0715, -80.4443) -> (23.0879, -80.498)
  line L579 (23.0879, -80.498) -> (23.1062, -80.551)
  line L580 (23.1062, -80.551) -> (23.1263, -80.6034)
  line L581 (23.1263, -80.6034) -> (23.1482, -80.6551)
  line L582 (23.1482, -80.6551) -> (23.172, -80.706)
  line L583 (23.172, -80.706) -> (23.1974, -80.756)
  line L584 (23.1974, -80.756) -> (23.2247, -80.8051)
  line L585 (23.2247, -80.8051) -> (23.2536, -80.8532)
  line L586 (23.2536, -80.8532) -> (23.2841, -80.9003)
  line L587 (23.2841, -80.9003) -> (23.3163, -80.9462)
  line L588 (23.3163, -80.9462) -> (23.3501, -80.9911)
  line L589 (23.3501, -80.9911) -> (23.3854, -81.0347)
  line L590 (23.3854, -81.0347) -> (23.4223, -81.0771)
  line L591 (23.4223, -81.0771) -> (23.4605, -81.1181)
  line L592 (23.4605, -81.1181) -> (23.5002, -81.1578)
  line L593 (23.5002, -81.1578) -> (23.5413, -81.1961)
  line L594 (23.5413, -81.1961) -> (23.5836, -81.2329)
  line L595 (23.5836, -81.2329) -> (23.6273, -81.2682)
  line L596 (23.6273, -81.2682) -> (23.6721, -81.302)
  line L597 (23.6721, -81.302) -> (23.7181, -81.3342)
  line L598 (23.7181, -81.3342) -> (23.7651, -81.3648)
  line L599 (23.7651, -81.3648) -> (23.8133, -81.3937)
  line L600 (23.8133, -81.3937) -> (23.8624, -81.4209)
  line L601 (23.8624, -81.4209) -> (23.9124, -81.4464)
  line L602 (23.9124, -81.4464) -> (23.9632, -81.4701)
  line L603 (23.9632, -81.4701) -> (24.0149, -81.492)
  line L604 (24.0149, -81.492) -> (24.0673, -81.5122)
  line L605 (24.0673, -81.5122) -> (24.1204, -81.5304)
  line L606 (24.1204, -81.5304) -> (24.1741, -81.5468)
  line L607 (24.1741, -81.5468) -> (24.2283, -81.5614)
  line L608 (24.2283, -81.5614) -> (24.283, -81.574)
  line L609 (24.283, -81.574) -> (24.3381, -81.5847)
  line L610 (24.3381, -81.5847) -> (24.3935, -81.5935)
  line L611 (24.3935, -81.5935) -> (24.4492, -81.6003)
  line L612 (24.4492, -81.6003) -> (24.5051, -81.6052)
  line L613 (24.5051, -81.6052) -> (24.5612, -81.6082)
  line L614 (24.5612, -81.6082) -> (24.6173, -81.6091)
  line L615 (24.6173, -81.6091) -> (24.673, -81.6082)
  line L616 (24.673, -81.6082) -> (24.7287, -81.6053)
  line L617 (24.7287, -81.6053) -> (24.7842, -81.6005)
  line L618 (24.7842, -81.6005) -> (24.8395, -81.5937)
  line L619 (24.8395, -81.5937) -> (24.8945, -81.5851)
  line L620 (24.8945, -81.5851) -> (24.9492, -81.5745)
  line L621 (24.9492, -81.5745) -> (25.0035, -81.5621)
  line L622 (25.0035, -81.5621) -> (25.0574, -81.5477)
  line L623 (25.0574, -81.5477) -> (25.1107, -81.5316)
  line L624 (25.1107, -81.5316) -> (25.1634, -81.5136)
  line L625 (25.1634, -81.5136) -> (25.2155, -81.4937)
  line L626 (25.2155, -81.4937) -> (25.2669, -81.4721)
  line L627 (25.2669, -81.4721) -> (25.3174, -81.4487)
  line L628 (25.3174, -81.4487) -> (25.3672, -81.4236)
  line L629 (25.3672, -81.4236) -> (25.416, -81.3968)
  line L630 (25.416, -81.3968) -> (25.4639, -81.3683)
  line L631 (25.4639, -81.3683) -> (25.5107, -81.3381)
  line L632 (25.5107, -81.3381) -> (25.5565, -81.3064)
  line L633 (25.5565, -81.3064) -> (25.6012, -81.273)
  line L634 (25.6012, -81.273) -> (25.6446, -81.2382)
  line L635 (25.6446, -81.2382) -> (25.6869, -81.2019)
  line L636 (25.6869, -81.2019) -> (25.7278, -81.1641)
  line L637 (25.7278, -81.1641) -> (25.7675, -81.1249)
  line L638 (25.7675, -81.1249) -> (25.8057, -81.0844)
  line L639 (25.8057, -81.0844) -> (25.8425, -81.0426)
  line L640 (25.8425, -81.0426) -> (25.8779, -80.9995)
  line L641 (25.8779, -80.9995) -> (25.9117, -80.9552)
  line L642 (25.9117, -80.9552) -> (25.944, -80.9098)
  line L643 (25.944, -80.9098) -> (25.9747, -80.8633)
  line L644 (25.9747, -80.8633) -> (26.0037, -80.8158)
  line L645 (26.0037, -80.8158) -> (26.0311, -80.7673)
  line L646 (26.0311, -80.7673) -> (26.0568, -80.7178)
  line L647 (26.0568, -80.7178) -> (26.0808, -80.6675)
  line L648 (26.0808, -80.6675) -> (26.103, -80.6164)
  line L649 (26.103, -80.6164) -> (26.1234, -80.5646)
  line L650 (26.1234, -80.5646) -> (26.142, -80.5121)
  line L651 (26.142, -80.5121) -> (26.1588, -80.4589)
  line L652 (26.1588, -80.4589) -> (26.1738, -80.4053)
  line L653 (26.1738, -80.4053) -> (26.1868, -80.3511)
  line L654 (26.1868, -80.3511) -> (26.198, -80.2965)
  line L655 (26.198, -80.2965) -> (26.2073, -80.2416)
  line L656 (26.2073, -80.2416) -> (26.2147, -80.1864)
  line L657 (26.2147, -80.1864) -> (26.2202, -80.1309)
  line L658 (26.2202, -80.1309) -> (26.2237, -80.0753)
  line L659 (26.2237, -80.0753) -> (26.2253, -80.0196)
  line L660 (26.2253, -80.0196) -> (26.225, -79.9639)
  line L661 (26.225, -79.9639) -> (26.2227, -79.9082)
  line L662 (26.2227, -79.9082) -> (26.2185, -79.8527)
  line L663 (26.2185, -79.8527) -> (26.2124, -79.7973)
  line L664 (26.2124, -79.7973) -> (26.2044, -79.7421)
  line L665 (26.2044, -79.7421) -> (26.1945, -79.6873)
  line L666 (26.1945, -79.6873) -> (26.1827, -79.6329)
  line L667 (26.1827, -79.6329) -> (26.169, -79.5788)
  line L668 (26.169, -79.5788) -> (26.1534, -79.5253)
  line L669 (26.1534, -79.5253) -> (26.136, -79.4724)
  line L670 (26.136, -79.4724) -> (26.1168, -79.4201)
  line L671 (26.1168, -79.4201) -> (26.0958, -79.3685)
  line L672 (26.0958, -79.3685) -> (26.073, -79.3177)
  line L673 (26.073, -79.3177) -> (26.0484, -79.2677)
  line L674 (26.0484, -79.2677) -> (26.0222, -79.2185)
  line L675 (26.0222, -79.2185) -> (25.9942, -79.1703)
  line L676 (25.9942, -79.1703) -> (25.9646, -79.1231)
  line L677 (25.9646, -79.1231) -> (25.9334, -79.077)
  line L678 (25.9334, -79.077) -> (25.9006, -79.0319)
  line L679 (25.9006, -79.0319) -> (25.8663, -78.9881)
  line L680 (25.8663, -78.9881) -> (25.8304, -78.9454)
  line L681 (25.8304, -78.9454) -> (25.7931, -78.904)
  line L682 (25.7931, -78.904) -> (25.7544, -78.8639)
  line L683 (25.7544, -78.8639) -> (25.7143, -78.8252)
  line L684 (25.7143, -78.8252) -> (25.6729, -78.7879)
  line L685 (25.6729, -78.7879) -> (25.6303, -78.7521)
  line L686 (25.6303, -78.7521) -> (25.5864, -78.7177)
  line L687 (25.5864, -78.7177) -> (25.5414, -78.6849)
  line L688 (25.5414, -78.6849) -> (25.4952, -78.6537)
  line L689 (25.4952, -78.6537) -> (25.448, -78.6241)
  line L690 (25.448, -78.6241) -> (25.3998, -78.5962)
  line L691 (25.3998, -78.5962) -> (25.3507, -78.5699)
  line L692 (25.3507, -78.5699) -> (25.3007, -78.5453)
  line L693 (25.3007, -78.5453) -> (25.2498, -78.5225)
  line L694 (25.2498, -78.5225) -> (25.1982, -78.5015)
  line L695 (25.1982, -78.5015) -> (25.1459, -78.4823)
  line L696 (25.1459, -78.4823) -> (25.093, -78.4649)
  line L697 (25.093, -78.4649) -> (25.0395, -78.4493)
  line L698 (25.0395, -78.4493) -> (24.9855, -78.4356)
  line L699 (24.9855, -78.4356) -> (24.931, -78.4238)
  line L700 (24.931, -78.4238) -> (24.8762, -78.4139)
  line L701 (24.8762, -78.4139) -> (24.8211, -78.4059)
  line L702 (24.8211, -78.4059) -> (24.7657, -78.3998)
  line L703 (24.7657, -78.3998) -> (24.7101, -78.3956)
  line L704 (24.7101, -78.3956) -> (24.6545, -78.3934)
  line L705 (24.6545, -78.3934) -> (24.5987, -78.393)
  line L706 (24.5987, -78.393) -> (24.543, -78.3946)
  line L707 (24.543, -78.3946) -> (24.4874, -78.3982)
  line L708 (24.4874, -78.3982) -> (24.432, -78.4036)
  line L709 (24.432, -78.4036) -> (24.3768, -78.411)
  line L710 (24.3768, -78.411) -> (24.3218, -78.4203)
  line L711 (24.3218, -78.4203) -> (24.2672, -78.4315)
  line L712 (24.2672, -78.4315) -> (24.2131, -78.4446)
  line L713 (24.2131, -78.4446) -> (24.1594, -78.4595)
  line L714 (24.1594, -78.4595) -> (24.1063, -78.4763)
  line L715 (24.1063, -78.4763) -> (24.0538, -78.4949)
  line L716 (24.0538, -78.4949) -> (24.0019, -78.5153)
  line L717 (24.0019, -78.5153) -> (23.9508, -78.5376)
  line L718 (23.9508, -78.5376) -> (23.9005, -78.5615)
  line L719 (23.9005, -78.5615) -> (23.8511, -78.5872)
  line L720 (23.8511, -78.5872) -> (23.8026, -78.6146)
  line L721 (23.8026, -78.6146) -> (23.755, -78.6437)
  line L722 (23.755, -78.6437) -> (23.7085, -78.6744)
  line L723 (23.7085, -78.6744) -> (23.6631, -78.7066)
  line L724 (23.6631, -78.7066) -> (23.6188, -78.7405)
  line L725 (23.6188, -78.7405) -> (23.5758, -78.7758)
  line L726 (23.5758, -78.7758) -> (23.5339, -78.8126)
  line L727 (23.5339, -78.8126) -> (23.4934, -78.8509)
  line L728 (23.4934, -78.8509) -> (23.4542, -78.8905)
  line L729 (23.4542, -78.8905) -> (23.4165, -78.9315)
  line L730 (23.4165, -78.9315) -> (23.3801, -78.9737)
  line L731 (23.3801, -78.9737) -> (23.3453, -79.0172)
  line L732 (23.3453, -79.0172) -> (23.312, -79.0618)
  line L733 (23.312, -79.0618) -> (23.2802, -79.1076)
  line L734 (23.2802, -79.1076) -> (23.2501, -79.1545)
  line L735 (23.2501, -79.1545) -> (23.2216, -79.2024)
  line L736 (23.2216, -79.2024) -> (23.1947, -79.2512)
  line L737 (23.1947, -79.2512) -> (23.1696, -79.3009)
  line L738 (23.1696, -79.3009) -> (23.1462, -79.3515)
  line L739 (23.1462, -79.3515) -> (23.1246, -79.4028)
  line L740 (23.1246, -79.4028) -> (23.1048, -79.4549)
  line L741 (23.1048, -79.4549) -> (23.0868, -79.5076)
  line L742 (23.0868, -79.5076) -> (23.0706, -79.561)
  line L743 (23.0706, -79.561) -> (23.0563, -79.6148)
  line L744 (23.0563, -79.6148) -> (23.0438, -79.6691)
  line L745 (23.0438, -79.6691) -> (23.0333, -79.7238)
  line L746 (23.0333, -79.7238) -> (23.0246, -79.7789)
  line L747 (23.0246, -79.7789) -> (23.0179, -79.8342)
  line L748 (23.0179, -79.8342) -> (23.0131, -79.8897)
  line L749 (23.0131, -79.8897) -> (23.0102, -79.9453)
  line L750 (23.0102, -79.9453) -> (23.0092, -80.001)
  circle A0 centre (24.5426, -79.9453) radius 1.4214
  circle A1 centre (52.5357, -79.9732) radius 1.4441
  circle A2 centre (19.5197, -27.9599) radius 1.4236
  circle A3 centre (67.7821, -29.1714) radius 1.4664
  point P0 (0, 0)
  constraints: 1502 end point, 4 centre point
extrude "Выдавливание7" cut sketch "Эскиз7" against normal blind 5.25 contours A0 | A1 | A2 | A3
fillet "Сопряжение4" [suppressed]
sketch "Эскиз8" plane through (-2, -96, 38) normal (-1, 0, 0) x (0, 0, 1)
  line L0 (-36, 103) -> (-36, 2.5093) projected
  line L1 (2, 2.5093) -> (2, 103) projected
  line L2 (-36, 14) -> (2, 14)
  line L3 (2, 14) -> (2, 89)
  line L4 (2, 89) -> (-36, 89)
  line L5 (-36, 89) -> (-36, 14)
  point P0 (-38, 96)
  dimension "d38" = 75
  constraints: 8 end point, 2 parallel, 1 horizontal, 1 perpendicular
  measures "d38" distance of L3.end L2.end
extrude "Выдавливание8" cut sketch "Эскиз8" against normal blind 92.25
